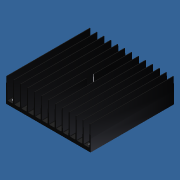
# Autodesk Inventor part: J002450
Saved by Autodesk Inventor 2015 SP1 (Build 190203100, 203)
## iProperties
Created: 2013-07-15
Material: ALUMINUM, 6061-T651
Vendor: HHMI: JFRC - ID&F
Document SubType Name: Modeling
Designer: NEGRASHOVI
Density: 2.7 g/cm^3
Mass: 861.061 g
Surface Area: 2240.49 cm^2
Volume: 318.912 cm^3
Project: P-129001
Description: HEAT SINK EXTRUSION ALTERED
Part Number: J002450
Appearance: Glossy - Black
RuleStatus: InUse
AfterDocSave0: file://Part Number Cleaner
LAB/DEPT: RUBIN (LAB)
REQUESTING SCIENTIST: ASO, YOSHI
SURFACE ROUGHNESS: N/A
DESIGN DEPARTMENT: HHMI: JRC - ID&F
SPECIAL FINISH: ANODIZE PER MIL-A-8625F, TYPE II, CLASS 2 (BLACK)
ALTERED ITEM PART NUMBER: 93H3803
ALTERED ITEM VENDOR: NEWARK (WWW.NEWARK.COM)
ALTERED ITEM DESCRIPTION: HEAT SINK EXTRUSION
Author: NEGRASHOVI
Revision Number: -
Autodesk Inventor part; units mm, degrees
ref_plane "YZ Plane" through (0, 0, 0) normal (1, 0, 0) x (0, 1, 0)
ref_plane "XZ Plane" through (0, 0, 0) normal (0, 1, 0) x (-1, 0, 0)
ref_plane "XY Plane" through (0, 0, 0) normal (0, 0, 1) x (1, 0, 0)
sketch "Sketch1" plane through (0, 0, 0) normal (0, 0, 1) x (1, 0, 0)
  line L0 (-88.9, -3.175) -> (88.9, -3.175)
  line L1 (88.9, -3.175) -> (88.9, 3.175)
  line L2 (88.9, 3.175) -> (-88.9, 3.175)
  line L3 (-88.9, 3.175) -> (-88.9, -3.175)
  line L4 (-88.9, -3.175) -> (88.9, 3.175) construction
  point P0 (0, 0)
  point P1 (0, 0)
  dimension "d0" = 6.35
  dimension "d1" = 177.8
  constraints: 10 end point, 2 parallel, 1 coincident, 1 horizontal, 1 midpoint, 1 perpendicular
  measures "d0" distance of L2.end L0.start
  measures "d1" distance of L0.start L0.end
extrude "Extrusion1" add sketch "Sketch1" against normal blind 152.4
sketch "Sketch2" plane through (0, 0, 0) normal (0, 0, 1) x (1, 0, 0)
  line L0 (88.9, 3.175) -> (-88.9, 3.175) projected
  line L1 (-77.47, 3.175) -> (-76.835, 41.275)
  line L2 (-76.835, 41.275) -> (-75.565, 41.275)
  line L3 (-75.565, 41.275) -> (-74.93, 3.175)
  line L4 (-74.93, 3.175) -> (-77.47, 3.175)
  line L5 (-76.2, 41.275) -> (-76.2, 3.175) construction
  point P0 (0, 0)
  dimension "d4" = 38.1
  dimension "d5" = 1.27
  dimension "d6" = 2.54
  dimension "d7" = 76.2
  constraints: 10 end point, 2 midpoint, 2 point on line, 1 collinear, 1 parallel, 1 vertical
  measures "d4" distance between parallel lines of L2 L0
  measures "d5" distance of L1.end L2.end
  measures "d6" distance of L3.end L1.start
  measures "d7" distance from line of point (0, 0) L5
extrude "Extrusion2" add sketch "Sketch2" against normal up to surface (152.4 mm away)
fillet "Fillet1" radius 1.27 2 edges at (-74.93, 3.175, -76.2) (-77.47, 3.175, -76.2)
full round fillet "Fillet2" first side at (-75.1555, 16.7076, -50.8) centre faces at (-75.9883, 41.275, -50.8) second side at (-77.0397, 28.9913, -50.8)
pattern_linear "Rectangular Pattern1" count 13 spacing 12.7 along (1, 0, 0) of "Extrusion2", "Fillet1", "Fillet2"
sketch "Sketch3" plane through (0, 0, 0) normal (0, 0, 1) x (1, 0, 0)
  line L0 (-88.9, -3.175) -> (88.9, -3.175) projected
  line L1 (-88.9, 3.175) -> (-88.9, -3.175) projected
  line L2 (-88.9, -3.175) -> (-77.216, -3.175)
  line L3 (-77.216, -3.175) -> (-77.216, 47.625)
  line L4 (-77.216, 47.625) -> (-88.9, 47.625)
  line L5 (-88.9, 47.625) -> (-88.9, -3.175)
  line L6 (0, -13.335) -> (0, 57.785) construction
  line L7 (88.9, -3.175) -> (77.216, -3.175)
  line L8 (77.216, -3.175) -> (77.216, 47.625)
  line L9 (77.216, 47.625) -> (88.9, 47.625)
  line L10 (88.9, 47.625) -> (88.9, -3.175)
  point P0 (0, 0)
  dimension "d14" = 50.8
  dimension "d15" = 154.432
  constraints: 16 end point, 3 symmetric about line, 2 parallel, 1 horizontal, 1 perpendicular
  measures "d14" distance of L4.end L0.start
  measures "d15" distance between parallel lines of L8 L3
extrude "Extrusion3" cut sketch "Sketch3" against normal through all
sketch "Sketch4" plane through (-77.216, -3.175, 0) normal (0, -1, 0) x (1, 0, 0)
  line L0 (0, 0) -> (154.432, 0) projected
  line L1 (154.432, -152.4) -> (154.432, 0) projected
  line L2 (0, -152.4) -> (154.432, -152.4) projected
  line L3 (0, 0) -> (0, -152.4) projected
  line L4 (77.216, 0) -> (77.216, -152.4) construction
  line L5 (0, -76.2) -> (154.432, -76.2) construction
  line L6 (7.366, -6.35) -> (147.066, -6.35) construction
  line L7 (147.066, -6.35) -> (147.066, -146.05) construction
  line L8 (147.066, -146.05) -> (7.366, -146.05) construction
  line L9 (7.366, -146.05) -> (7.366, -6.35) construction
  line L10 (115.316, -38.1) -> (39.116, -38.1) construction
  line L11 (39.116, -38.1) -> (39.116, -114.3) construction
  line L12 (39.116, -114.3) -> (115.316, -114.3) construction
  line L13 (115.316, -114.3) -> (115.316, -38.1) construction
  line L14 (89.916, -62.23) -> (64.516, -62.23) construction
  line L15 (64.516, -62.23) -> (64.516, -90.17) construction
  line L16 (64.516, -90.17) -> (89.916, -90.17) construction
  line L17 (89.916, -90.17) -> (89.916, -62.23) construction
  line L18 (115.316, -38.1) -> (39.116, -114.3) construction
  line L19 (89.916, -62.23) -> (64.516, -90.17) construction
  point P0 (77.216, -76.2)
  point P1 (7.366, -6.35)
  point P2 (147.066, -6.35)
  point P3 (77.216, -76.2)
  dimension "d25" = 139.7
  dimension "d26" = 139.7
  dimension "d34" = 76.2
  dimension "d35" = 76.2
  dimension "d36" = 25.4
  dimension "d37" = 27.94
  constraints: 32 end point, 12 coincident, 7 midpoint, 6 parallel, 3 horizontal, 3 perpendicular, 2 other
  measures "d25" distance of L6.start L6.end
  measures "d26" distance of L8.end L6.start
  measures "d34" distance of L10.end L11.end
  measures "d35" distance of L10.start L10.end
  measures "d36" distance of L14.start L14.end
  measures "d37" distance of L14.end L15.end
hole "Hole1" at (0, -3.175, -76.2) direction (0, 1, 0) diameter 7.62 end through all
hole "Hole2" at (-69.85, -3.175, -6.35) at (69.85, -3.175, -6.35) at (69.85, -3.175, -146.05) at (-69.85, -3.175, -146.05) direction (0, 1, 0) diameter 3.81 end through all clearance for "Flat Head Machine Screw (82)" size "#6" standard "Ansi Unified Screw Threads"
sketch "Sketch5" plane through (2.519, 3.175, 0) normal (0, 1, 0) x (1, 0, 0)
  circle A0 centre (-2.519, 76.2) radius 6.35
  point P0 (-2.519, 0)
  point P1 (-72.369, 146.05)
  point P2 (67.331, 146.05)
  point P3 (67.331, 6.35)
  point P4 (-72.369, 6.35)
  dimension "d45" = 12.7
  constraints: 1 centre point, 1 coincident
  measures "d45" diameter of A0
extrude "Extrusion4" cut sketch "Sketch5" along normal blind 50.8 and the other way blind 0.254
equation "\"d26\" = d25"
body "Solid1"
